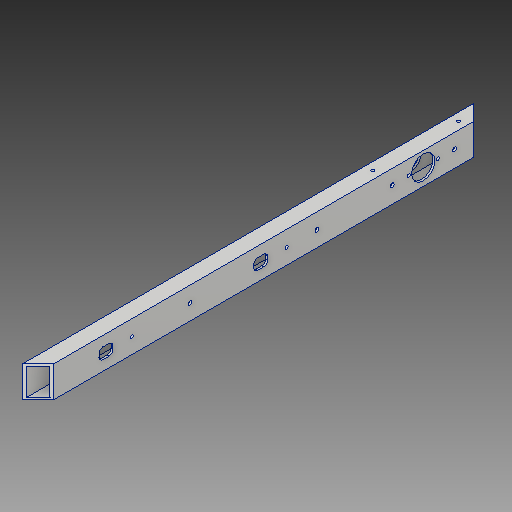
# Autodesk Inventor part: FRA_MainRail_001
Saved by Autodesk Inventor 2018.3 (Build 223284000, 284)
## iProperties
Created: 2020-01-08
Part Number: FRA_MainRail_001
Material: Aluminum 6061
Document SubType Name: Modeling
Designer: user
Mass: 814.413 g
Surface Area: 1940.98 cm^2
Volume: 301.634 cm^3
Density: 2.7 g/cm^3
Appearance: Aluminum - Flat
Author: user
Autodesk Inventor part; units mm, degrees
sketch "Sketch1" plane through (0, 0, 0) normal (0, 0, 1) x (1, 0, 0)
  line L0 (0, 0) -> (25.4, 0)
  line L1 (25.4, 0) -> (25.4, 50.8)
  line L2 (25.4, 50.8) -> (0, 50.8)
  line L3 (0, 50.8) -> (0, 0)
  line L4 (3.175, 3.175) -> (22.225, 3.175)
  line L5 (22.225, 3.175) -> (22.225, 47.625)
  line L6 (22.225, 47.625) -> (3.175, 47.625)
  line L7 (3.175, 47.625) -> (3.175, 3.175)
  dimension "d0" = 25.4
  dimension "d1" = 50.8
  dimension "d2" = 3.175
  constraints: 16 end point, 4 parallel, 2 perpendicular, 1 horizontal, 3 other
  measures "d0" distance of L2.end L1.end
  measures "d1" distance of L1.end L0.end
  measures "d2" distance between parallel lines of L3 L7
extrude "Extrusion1" add sketch "Sketch1" along normal mid plane 736.6
chamfer "Chamfer1" distance 25.4 angle 45 2 edges at (25.4, 25.4, 368.3) (25.4, 25.4, -368.3)
sketch "Sketch2" plane through (0, 50.8, 368.3) normal (0, 1, 0) x (1, 0, 0)
  line L0 (1.3146, 262.6687) -> (16.4951, 262.6687) construction
  line L1 (16.4951, 262.6687) -> (16.4951, 100.7429) construction
  line L2 (16.4951, 100.7429) -> (1.3146, 100.7429) construction
  line L3 (1.3146, 100.7429) -> (1.3146, 262.6687) construction
  point P0 (0, 368.3)
  constraints: 2 other
sketch "Sketch3" plane through (25.4, 0, -342.9) normal (1, 0, 0) x (0, 0, -1)
  line L0 (0, 50.8) -> (0, 0) projected
  line L1 (0, 50.8) -> (-685.8, 50.8) projected
  line L2 (-685.8, 0) -> (-685.8, 50.8) projected
  line L3 (0, 0) -> (-685.8, 0) projected
  line L4 (-342.9, -10.16) -> (-342.9, 60.96) projected
  point P0 (-342.9, 0)
  point P1 (-82.55, 26.9875)
  dimension "d8" = 685.8
  dimension "d79" = 26.9875
  dimension "d80" = 260.35
  measures "d8" distance of L0.start L1.end
  measures "d79" distance from line of L3 point (-82.55, 26.988)
  measures "d80" distance from line of L4 point (-82.55, 26.988)
ref_plane "Work Plane1" through (0, 25.4, 368.3) normal (0, 1, 0) x (1, 0, 0)
hole "Hole1" at (25.4, 26.9875, -260.35) direction (-1, 0, 0) diameter 38.1 end through all
sketch "Sketch4" plane through (25.4, 0, -342.9) normal (1, 0, 0) x (0, 0, -1)
  circle A0 centre (-82.55, 26.9875) radius 19.05 projected
  line L0 (0, 50.8) -> (0, 0) projected
  line L1 (0, 50.8) -> (-685.8, 50.8) projected
  line L2 (-685.8, 0) -> (-685.8, 50.8) projected
  line L3 (0, 0) -> (-685.8, 0) projected
  point P0 (-342.9, 0)
  point P1 (-106.3625, 26.9875)
  point P2 (-58.7375, 26.9875)
  dimension "d81" = 26.9875
  dimension "d82" = 26.9875
  dimension "d83" = 23.8125
  dimension "d84" = 23.8125
  measures "d81" distance from line of L3 point (-106.362, 26.988)
  measures "d82" distance from line of L3 point (-58.737, 26.988)
  measures "d83" distance of A0.centre point (-58.737, 26.988)
  measures "d84" distance of A0.centre point (-106.362, 26.988)
hole "Hole2" at (25.4, 26.9875, -284.1625) at (25.4, 26.9875, -236.5375) direction (-1, 0, 0) diameter 5.1054 end through all
ref_plane "Work Plane4" through (-713.3864, 26.9875, -236.5375) normal (0, 1, 0) x (1, 0, 0)
ref_plane "Work Plane2" through (-713.3864, 26.9875, -236.5375) normal (0, 1, 0) x (1, 0, 0)
sketch "Sketch5" plane through (25.4, 0, -342.9) normal (1, 0, 0) x (0, 0, -1)
  line L0 (-353.0553, 16.4846) -> (-342.9207, 16.4846)
  line L1 (-336.5707, 22.8346) -> (-336.5707, 27.9654)
  line L2 (-342.9207, 34.3154) -> (-353.0553, 34.3154)
  line L3 (-359.4053, 27.9654) -> (-359.4053, 22.8346)
  line L4 (0, 50.8) -> (-685.8, 50.8) projected
  circle A0 centre (-58.7375, 26.9875) radius 2.5527 projected
  circle A1 centre (-106.3625, 26.9875) radius 2.5527 projected
  circle A2 centre (-82.55, 26.9875) radius 19.05 projected
  line L5 (0, 50.8) -> (0, 0) projected
  line L6 (0, 50.8) -> (-685.8, 50.8) projected
  line L7 (-685.8, 0) -> (-685.8, 50.8) projected
  line L8 (0, 0) -> (-685.8, 0) projected
  arc A3 (-353.0553, 34.3154) -> (-359.4053, 27.9654) centre (-353.0553, 27.9654) ccw
  arc A4 (-336.5707, 27.9654) -> (-342.9207, 34.3154) centre (-342.9207, 27.9654) ccw
  arc A5 (-359.4053, 22.8346) -> (-353.0553, 16.4846) centre (-353.0553, 22.8346) ccw
  arc A6 (-342.9207, 16.4846) -> (-336.5707, 22.8346) centre (-342.9207, 22.8346) ccw
  line L9 (-858.52, 26.9875) -> (172.72, 26.9875) projected
  line L10 (-342.9, -10.16) -> (-342.9, 60.96) projected
  point P0 (-342.9, 0)
  point P1 (-359.4053, 16.4846)
  point P2 (-336.5707, 34.3154)
  point P3 (-359.4053, 34.3154)
  point P4 (-350.0327, 25.4)
  dimension "d38" = 6.35
  dimension "d88" = 685.8
  dimension "d89" = 82.55
  dimension "d119" = 267.4874
  dimension "d132" = 17.8308
  dimension "d134" = 25.4
  dimension "d135" = 8.9154
  dimension "d136" = 9.3726
  dimension "d146" = 13.462
  dimension "d147" = 22.8346
  constraints: 8 end point, 8 point on circle, 8 tangent, 6 point on line, 4 centre point, 3 equal radius, 2 parallel, 1 horizontal, 1 perpendicular
  measures "d38" radius of A3
  measures "d88" distance of L5.start L6.end
  measures "d89" distance from line of L5 A2.centre
  measures "d119" distance of point (-350.033, 25.4) A2.centre
  measures "d132" distance between parallel lines of L0 L2
  measures "d134" distance from line of L4 point (-350.033, 25.4)
  measures "d135" distance from line of L2 point (-350.033, 25.4)
  measures "d136" distance from line of L3 point (-350.033, 25.4)
  measures "d146" distance from line of L1 point (-350.033, 25.4)
  measures "d147" distance between parallel lines of L3 L1
extrude "Extrusion2" cut sketch "Sketch5" against normal blind 50.8 contours A5 L3 L9 L10 A6 L0 | L10 L9 L1 A6 | L3 A3 L2 A4 L10 L9 | L10 A4 L1 L9
sketch "Sketch6" plane through (25.4, 0, -342.9) normal (1, 0, 0) x (0, 0, -1)
  line L0 (-353.0553, 34.3154) -> (-342.9207, 34.3154) projected
  circle A0 centre (-58.7375, 26.9875) radius 2.5527 projected
  circle A1 centre (-106.3625, 26.9875) radius 2.5527 projected
  circle A2 centre (-82.55, 26.9875) radius 19.05 projected
  line L1 (0, 50.8) -> (0, 0) projected
  line L2 (0, 50.8) -> (-685.8, 50.8) projected
  line L3 (-685.8, 0) -> (-685.8, 50.8) projected
  line L4 (0, 0) -> (-685.8, 0) projected
  point P0 (-342.9, 0)
  point P1 (-305.7859, 25.4)
  point P2 (-127, 28.575)
  point P3 (-350.0327, 25.4)
  dimension "d66" = 25.4
  dimension "d137" = 44.2468
  measures "d66" distance from line of L4 point (-305.786, 25.4)
  measures "d137" distance of point (-305.786, 25.4) point (-350.033, 25.4)
hole "Hole3" at (25.4, 25.4, -37.1141) direction (-1, 0, 0) diameter 4.9784 end through all
sketch "Sketch10" plane through (25.4, 0, -342.9) normal (1, 0, 0) x (0, 0, -1)
  line L0 (-605.559, 16.4846) -> (-595.4244, 16.4846)
  line L1 (-589.0744, 22.8346) -> (-589.0744, 27.9654)
  line L2 (-595.4244, 34.3154) -> (-605.559, 34.3154)
  line L3 (-611.909, 27.9654) -> (-611.909, 22.8346)
  arc A0 (-605.559, 34.3154) -> (-611.909, 27.9654) centre (-605.559, 27.9654) ccw
  arc A1 (-589.0744, 27.9654) -> (-595.4244, 34.3154) centre (-595.4244, 27.9654) ccw
  arc A2 (-611.909, 22.8346) -> (-605.559, 16.4846) centre (-605.559, 22.8346) ccw
  arc A3 (-595.4244, 16.4846) -> (-589.0744, 22.8346) centre (-595.4244, 22.8346) ccw
  line L4 (-858.52, 26.9875) -> (172.72, 26.9875) projected
  line L5 (-342.9, -10.16) -> (-342.9, 60.96) projected
  circle A4 centre (-305.7859, 25.4) radius 2.4892 projected
  circle A5 centre (-58.7375, 26.9875) radius 2.5527 projected
  circle A6 centre (-106.3625, 26.9875) radius 2.5527 projected
  circle A7 centre (-82.55, 26.9875) radius 19.05 projected
  line L6 (0, 50.8) -> (0, 0) projected
  line L7 (0, 50.8) -> (-685.8, 50.8) projected
  line L8 (-685.8, 0) -> (-685.8, 50.8) projected
  line L9 (0, 0) -> (-685.8, 0) projected
  point P0 (-611.909, 16.4846)
  point P1 (-589.0744, 34.3154)
  point P2 (-611.909, 34.3154)
  point P3 (-602.5364, 25.4)
  dimension "d91" = 6.35
  dimension "d107" = 260.35
  dimension "d120" = 519.9888
  dimension "d138" = 17.8308
  dimension "d139" = 22.8346
  dimension "d140" = 25.4
  dimension "d141" = 8.9154
  dimension "d142" = 9.3726
  dimension "d148" = 3.0226
  dimension "d149" = 7.112
  constraints: 8 end point, 8 point on circle, 8 tangent, 6 point on line, 4 centre point, 3 equal radius, 2 parallel, 1 horizontal, 1 perpendicular
  measures "d91" radius of A0
  measures "d107" distance from line of A7.centre L5
  measures "d120" distance of A7.centre point (-602.536, 25.4)
  measures "d138" distance between parallel lines of L0 L2
  measures "d139" distance between parallel lines of L3 L1
  measures "d140" distance from line of L7 point (-602.536, 25.4)
  measures "d141" distance from line of L2 point (-602.536, 25.4)
  measures "d142" distance from line of L3 point (-602.536, 25.4)
  measures "d148" horizontal distance of point (-602.536, 25.4) A0.centre
  measures "d149" horizontal distance of A1.centre point (-602.536, 25.4)
extrude "Extrusion3" cut sketch "Sketch10" against normal through all contours A2 L3 L4 L1 A3 L0 | L3 A0 L2 A1 L1 L4
sketch "Sketch11" plane through (25.4, 0, -342.9) normal (1, 0, 0) x (0, 0, -1)
  line L0 (0, 50.8) -> (-685.8, 50.8) projected
  circle A0 centre (-305.7859, 25.4) radius 2.4892 projected
  line L1 (-611.909, 22.8346) -> (-611.909, 27.9654) projected
  point P0 (-342.9, 0)
  point P1 (-558.2896, 25.4)
  point P2 (-602.5364, 25.4)
  dimension "d110" = 25.4
  dimension "d143" = 44.2468
  measures "d110" distance from line of L0 point (-558.29, 25.4)
  measures "d143" distance of point (-558.29, 25.4) point (-602.536, 25.4)
hole "Hole4" at (25.4, 25.4, 215.3896) direction (-1, 0, 0) diameter 4.9784 end through all
sketch "Sketch12" plane through (25.4, 0, -342.9) normal (1, 0, 0) x (0, 0, -1)
  line L0 (0, 0) -> (-685.8, 0) projected
  circle A0 centre (-558.2896, 25.4) radius 2.4892 projected
  circle A1 centre (-305.7859, 25.4) radius 2.4892 projected
  circle A2 centre (-58.7375, 26.9875) radius 2.5527 projected
  circle A3 centre (-106.3625, 26.9875) radius 2.5527 projected
  circle A4 centre (-82.55, 26.9875) radius 19.05 projected
  line L1 (0, 50.8) -> (0, 0) projected
  line L2 (0, 50.8) -> (-685.8, 50.8) projected
  line L3 (-685.8, 0) -> (-685.8, 50.8) projected
  line L4 (0, 0) -> (-685.8, 0) projected
  point P0 (-342.9, 0)
  point P1 (-133.35, 26.9875)
  point P2 (-31.75, 26.9875)
  dimension "d121" = 26.9875
  dimension "d122" = 50.8
  dimension "d123" = 50.8
  dimension "d124" = 26.9875
  measures "d121" distance from line of L0 point (-133.35, 26.988)
  measures "d122" distance of A4.centre point (-133.35, 26.988)
  measures "d123" distance of point (-31.75, 26.988) A4.centre
  measures "d124" distance from line of L4 point (-31.75, 26.988)
hole "Hole5" at (25.4, 26.9875, -209.55) at (25.4, 26.9875, -311.15) direction (-1, 0, 0) diameter 6.5278 end through all
sketch "Sketch13" plane through (25.4, 0, -342.9) normal (1, 0, 0) x (0, 0, -1)
  point P0 (-342.9, 0)
  point P1 (-350.0327, 25.4)
  point P2 (-305.7859, 25.4)
  dimension "d145" = 44.2468
  measures "d145" distance of point (-305.786, 25.4) point (-350.033, 25.4)
sketch "Sketch14" plane through (0, 50.8, 368.3) normal (0, 1, 0) x (1, 0, 0)
  line L0 (-18.949, 736.6) -> (42.0825, 736.6) construction
  line L1 (0, 736.6) -> (0, 0) construction
  point P0 (0, 368.3)
  point P1 (12.7, 698.5)
  point P2 (12.7, 558.8)
  dimension "d150" = 38.1
  dimension "d151" = 139.7
  dimension "d152" = 12.7
  constraints: 2 end point, 1 horizontal, 1 point on line, 1 vertical alignment
  measures "d150" distance from line of point (12.7, 698.5) L0
  measures "d151" distance of point (12.7, 558.8) point (12.7, 698.5)
  measures "d152" distance from line of L1 point (12.7, 698.5)
hole "Hole6" at (12.7, 50.8, -330.2) at (12.7, 50.8, -190.5) direction (0, -1, 0) diameter 5.1054 end through all clearance for "Flat Head Machine Screw (82)" size "#10" standard "Ansi Unified Screw Threads"
sketch "Sketch15" plane through (0, 0, 368.3) normal (-1, 0, 0) x (0, 0, 1)
  line L0 (0, 50.8) -> (0, 0) projected
  line L1 (-883.92, 26.9875) -> (147.32, 26.9875) projected
  line L2 (-883.92, 25.4) -> (147.32, 25.4) projected
  point P0 (-368.3, 0)
  point P1 (-454.9902, 25.4)
  point P2 (-247.65, 25.4)
  dimension "d161" = 454.9902
  dimension "d169" = 247.65
  constraints: 1 horizontal alignment, 1 point on line
  measures "d161" distance from line of L0 point (-454.99, 25.4)
  measures "d169" distance from line of L0 point (-247.65, 25.4)
hole "Hole8" at (0, 25.4, 120.65) at (0, 25.4, -86.6902) direction (1, 0, 0) diameter 6.35 end through all counterbore diameter 9.525 counterbore depth 12.7
equation "\"d84\" = d83"
body "Solid1"
